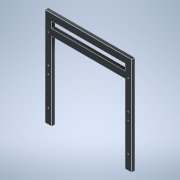
# Autodesk Inventor part: Base
Saved by Autodesk Inventor 2021 (Build 250183000, 183)
## iProperties
Created: 2022-01-26
Part Number: Base
Material: Hierro, fundido
Document SubType Name: Modeling
Designer: arthu
Density: 7.15 g/cm^3
Appearance: Gris hierro
Author: arthu
Autodesk Inventor part; units mm, degrees
ref_plane "YZ Plane" through (0, 0, 0) normal (1, 0, 0) x (0, 1, 0)
ref_plane "XZ Plane" through (0, 0, 0) normal (0, 1, 0) x (-1, 0, 0)
ref_plane "XY Plane" through (0, 0, 0) normal (0, 0, 1) x (1, 0, 0)
sketch "Boceto1" plane through (0, 0, 0) normal (0, 0, 1) x (1, 0, 0)
  line L0 (510, 575) -> (510, -575)
  line L1 (-510, -575) -> (-510, 575)
  line L2 (-510, 575) -> (510, -575) construction
  line L3 (510, 575) -> (-510, -575) construction
  line L4 (430, -495) -> (430, -575)
  line L5 (-430, -495) -> (-430, -575)
  line L6 (-510, 575) -> (-430, 575)
  line L7 (430, 575) -> (510, 575)
  line L8 (510, -575) -> (430, -575)
  line L9 (-430, -575) -> (-510, -575)
  line L10 (-430, 575) -> (430, 575)
  line L11 (430, 495) -> (-430, 495)
  line L12 (-430, 495) -> (-430, 420)
  line L13 (-430, 420) -> (430, 420)
  line L14 (-430, 340) -> (430, 340)
  line L15 (-430, 495) -> (-430, 420)
  line L16 (-430, 340) -> (-430, -495)
  line L17 (430, -495) -> (430, 340)
  line L18 (430, 420) -> (430, 495)
  line L19 (510, 0) -> (430, 0)
  line L20 (-430, 0) -> (-510, 0)
  point P0 (0, 0)
  point P1 (470, 0)
  point P2 (-470, 0)
  dimension "d0" = 1020
  dimension "d1" = 1150
  dimension "d18" = 940
  constraints: 42 end point, 11 perpendicular, 10 parallel, 6 midpoint, 3 horizontal, 3 point on line
  measures "d0" distance of L0.end L1.start
  measures "d1" distance of L0.start L0.end
  measures "d18" distance of point (470, 0) point (-470, 0)
extrude "Extrusión1" add sketch "Boceto1" along normal blind 40
shell "Vaciado1" thickness 2.5 removed faces 2 at (456.6667, -575, 13.3333) at (-483.3333, -575, 13.3333)
sketch "Boceto2" plane through (0, 0, 40) normal (0, 0, 1) x (1, 0, 0)
  line L0 (-510, -575) -> (-430, -575) projected
  line L1 (-470, -575) -> (-470, -405)
  circle A0 centre (-470, -405) radius 6.5
  line L2 (432.5, -575) -> (507.5, -575) projected
  line L3 (470, -575) -> (470, -405)
  circle A1 centre (470, -405) radius 6.5
  line L4 (-470, -405) -> (-470, 365)
  circle A2 centre (-470, 365) radius 6.5
  line L5 (470, -405) -> (470, 365)
  circle A3 centre (470, 365) radius 6.5
  point P0 (0, 0)
  dimension "d8" = 170
  dimension "d9" = 13
  dimension "d10" = 13
  dimension "d13" = 770
  dimension "d14" = 13
  dimension "d15" = 770
  dimension "d16" = 13
  constraints: 8 end point, 4 centre point, 4 coincident, 3 vertical, 2 midpoint, 1 point on line
  measures "d8" distance of L1.start L1.end
  measures "d9" diameter of A0
  measures "d10" diameter of A1
  measures "d13" distance of L4.start L4.end
  measures "d14" diameter of A2
  measures "d15" distance of L5.start L5.end
  measures "d16" diameter of A3
extrude "Extrusión2" cut sketch "Boceto2" against normal blind 100
fillet "Empalme1" radius 2 22 edges at (510, 0, 40) (0, 575, 40) (430, -117.5, 40) (0, 340, 40) (0, 420, 40) (430, 457.5, 40) (0, 495, 40) (-430, 457.5, 40) (-430, -117.5, 40) (-510, 0, 40) (-510, 0, 0) (-430, -117.5, 0) (0, 575, 0) (0, 495, 0) (0, 417.5, 2.5) (0, 340, 0) (430, -117.5, 0) (430, 457.5, 0) (-430, 457.5, 0) (-510, 575, 20) (510, 575, 20) (510, 0, 0)
sketch "Boceto3" plane through (0, 0, 0) normal (0, 0, -1) x (-1, 0, 0)
  point P0 (0, 0)
sketch "Boceto4" plane through (0, 0, 0) normal (0, 0, -1) x (-1, 0, 0)
  circle A0 centre (-470, 365) radius 6.5 projected
  circle A1 centre (-470, -405) radius 6.5 projected
  circle A2 centre (-470, 365) radius 6.5 projected
  circle A3 centre (-470, -405) radius 6.5 projected
  line L0 (-470, 365) -> (-470, -405)
  line L1 (-470, -20) -> (-470, 25.2)
  circle A4 centre (-470, 25.2) radius 6.5
  line L2 (-470, -20) -> (-470, -65.2)
  circle A5 centre (-470, -65.2) radius 6.5
  line L3 (0, 0) -> (0, -640.3726)
  circle A6 centre (470, 25.2) radius 6.5
  circle A7 centre (470, -65.2) radius 6.5
  circle A8 centre (470, 365) radius 6.5 projected
  circle A9 centre (470, -405) radius 6.5 projected
  line L4 (470, 365) -> (470, -405)
  line L5 (-470, 365) -> (-470, -20)
  point P0 (470, -20)
  point P1 (-470, -42.6)
  dimension "d19" = 45.2
  dimension "d20" = 13
  dimension "d21" = 45.2
  dimension "d22" = 13
  dimension "d25" = 45.2
  dimension "d26" = 385
  constraints: 12 end point, 4 centre point, 3 midpoint, 3 vertical, 2 coincident, 2 point on line, 2 symmetric about line, 1 collinear, 2 other
  measures "d19" distance of L1.start L1.end
  measures "d20" diameter of A4
  measures "d21" distance of L1.start L2.end
  measures "d22" diameter of A5
  measures "d25" distance of A6.centre point (470, -20)
  measures "d26" distance of L0.start L1.start
extrude "Extrusión3" cut sketch "Boceto4" against normal blind 100 contours A4 L0 | L0 A4 | A5 L0 | L0 A5 | A6 L4 | L4 A6 | A7 L4 | L4 A7
